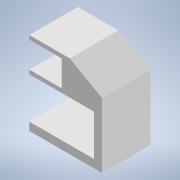
# Autodesk Inventor part: SwerveBracket
Saved by Autodesk Inventor 2022.3 (Build 263350000, 350)
## iProperties
Created: 2022-04-28
Part Number: SwerveBracket
Material: Generic
Document SubType Name: Modeling
Designer: Robert Nies
Density: 1 g/cm^3
Appearance: Default
Author: Robert Nies
Autodesk Inventor part; units mm, degrees
ref_plane "YZ Plane" through (0, 0, 0) normal (1, 0, 0) x (0, 1, 0)
ref_plane "XZ Plane" through (0, 0, 0) normal (0, 1, 0) x (-1, 0, 0)
ref_plane "XY Plane" through (0, 0, 0) normal (0, 0, 1) x (1, 0, 0)
sketch "Sketch1" plane through (0, 0, 0) normal (0, 0, 1) x (1, 0, 0)
  line L0 (2.6235, 11.5434) -> (28.0235, 11.5434)
  line L1 (28.0235, 11.5434) -> (28.0235, 14.7184)
  line L2 (28.0235, 14.7184) -> (2.6235, 14.7184)
  line L3 (2.6235, 14.7184) -> (2.6235, 11.5434)
  line L4 (28.0235, -8.7766) -> (2.6235, -8.7766)
  line L5 (2.6235, -8.7766) -> (2.6235, -11.9516)
  line L6 (2.6235, -11.9516) -> (28.0235, -11.9516)
  line L7 (28.0235, -11.9516) -> (28.0235, -8.7766)
  line L8 (28.0235, -11.9516) -> (34.3735, -11.9516)
  line L9 (34.3735, -11.9516) -> (34.3735, 14.7184)
  line L10 (34.3735, 14.7184) -> (28.0235, 14.7184)
  line L11 (28.0235, 14.7184) -> (28.0235, -11.9516)
  line L12 (2.6235, -50.4767) -> (53.4235, -50.4767)
  line L13 (53.4235, -50.4767) -> (53.4235, -44.1267)
  line L14 (53.4235, -44.1267) -> (2.6235, -44.1267)
  line L15 (2.6235, -44.1267) -> (2.6235, -50.4767)
  line L16 (53.4235, -50.4767) -> (59.7735, -50.4767)
  line L17 (59.7735, -50.4767) -> (59.7735, 0.3233)
  line L18 (59.7735, 0.3233) -> (53.4235, 0.3233)
  line L19 (53.4235, 0.3233) -> (53.4235, -50.4767)
  line L20 (34.3735, -11.9516) -> (53.4235, -11.9516)
  line L21 (59.7735, 0.3233) -> (34.3735, 14.7184)
  point P0 (0, 0)
  dimension "d0" = 25.4
  dimension "d1" = 3.175
  dimension "d2" = 3.175
  dimension "d3" = 20.32
  dimension "d4" = 6.35
  dimension "d5" = 50.8
  dimension "d6" = 6.35
  dimension "d7" = 6.35
  dimension "d8" = 50.8
  constraints: 44 end point, 10 parallel, 6 perpendicular, 5 horizontal, 3 point on line, 1 collinear
  measures "d0" distance of L2.end L1.end
  measures "d1" distance of L1.end L0.end
  measures "d2" distance of L5.end L4.end
  measures "d3" distance between parallel lines of L0 L4
  measures "d4" distance of L10.end L9.end
  measures "d5" distance of L14.end L13.end
  measures "d6" distance of L13.end L12.end
  measures "d7" distance of L18.end L17.end
  measures "d8" distance of L17.end L16.end
extrude "Extrusion1" add sketch "Sketch1" along normal blind 50.8
sketch "Sketch2" plane through (59.7735, -50.4767, 0) normal (1, 0, 0) x (0, 0, -1)
  circle A0 centre (-25.4, 25.4) radius 3.175
  line L0 (0, 50.8) -> (-50.8, 50.8) projected
  line L1 (-50.8, 0) -> (-50.8, 50.8) projected
  point P0 (0, 50.4767)
  dimension "d11" = 6.35
  dimension "d12" = 25.4
  dimension "d13" = 25.4
  constraints: 1 centre point
  measures "d11" diameter of A0
  measures "d12" distance from line of L0 A0.centre
  measures "d13" distance from line of L1 A0.centre
extrude "Extrusion2" cut sketch "Sketch2" against normal blind 25.4
sketch "Sketch3" plane through (2.6235, 14.7184, 0) normal (0, 1, 0) x (1, 0, 0)
  circle A0 centre (3.175, -6.35) radius 1.5875
  circle A1 centre (20.955, -6.35) radius 1.5875
  line L0 (31.75, 0) -> (0, 0) projected
  line L1 (0, 0) -> (0, -50.8) projected
  point P0 (-2.6235, 0)
  dimension "d16" = 3.175
  dimension "d17" = 3.175
  dimension "d18" = 6.35
  dimension "d19" = 6.35
  dimension "d20" = 17.78
  dimension "d21" = 3.175
  constraints: 2 centre point
  measures "d16" diameter of A0
  measures "d17" diameter of A1
  measures "d18" distance from line of L0 A1.centre
  measures "d19" distance from line of L0 A0.centre
  measures "d20" distance of A0.centre A1.centre
  measures "d21" distance from line of L1 A0.centre
extrude "Extrusion3" cut sketch "Sketch3" against normal blind 27.94
fillet "Fillet1" radius 3.175 7 edges at (34.3735, 14.7184, 25.4) (59.7735, 0.3233, 25.4) (59.7735, -50.4767, 25.4) (53.4235, -11.9516, 25.4) (53.4235, -44.1267, 25.4) (2.6235, -50.4767, 25.4) (2.6235, -44.1267, 25.4)
fillet "Fillet2" radius 0.508 6 edges at (2.6235, -8.7766, 25.4) (2.6235, -11.9516, 25.4) (2.6235, 11.5434, 25.4) (2.6235, 14.7184, 25.4) (28.0235, 11.5434, 25.4) (28.0235, -8.7766, 25.4)
equation "\"d14\" = d12"
body "Solid1"
